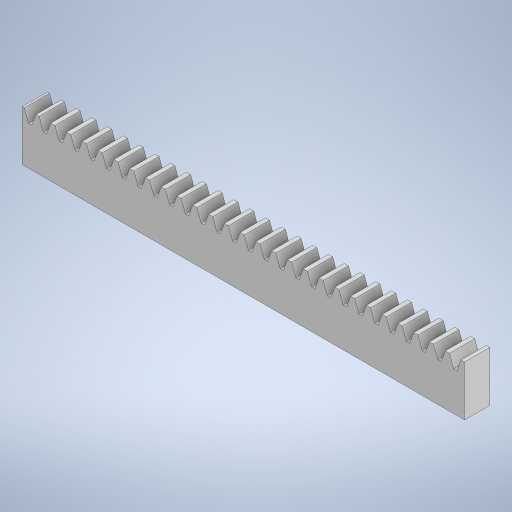
# Autodesk Inventor part: 래크수정
Saved by Autodesk Inventor 2024 (Build 280153000, 153)
## iProperties
Created: 2023-09-21
Part Number: 래크수정
Material: 일반
Document SubType Name: Modeling
Designer: user
Density: 1 g/cm^3
Appearance: 기본값
Author: user
Autodesk Inventor part; units mm, degrees
ref_plane "YZ Plane" through (0, 0, 0) normal (1, 0, 0) x (0, 1, 0)
ref_plane "XZ Plane" through (0, 0, 0) normal (0, 1, 0) x (-1, 0, 0)
ref_plane "XY Plane" through (0, 0, 0) normal (0, 0, 1) x (1, 0, 0)
sketch "스케치1" plane through (0, 0, 0) normal (0, 0, 1) x (1, 0, 0)
  line L0 (32.407, 33.8175) -> (32.407, 13.8175)
  line L1 (32.407, 13.8175) -> (-143.593, 13.8175)
  line L2 (-143.593, 13.8175) -> (-143.593, 33.8175)
  line L3 (-143.593, 29.3175) -> (32.407, 29.3175) construction
  line L4 (32.407, 31.8175) -> (-143.593, 31.8175) construction
  line L5 (-143.593, 29.8175) -> (32.407, 29.8175) construction
  line L6 (-140.453, 26.9927) -> (-140.453, 39.5951) construction
  line L7 (-137.313, 29.3175) -> (-137.313, 39.4326) construction
  line L8 (-142.751, 33.8175) -> (-141.1131, 29.3175)
  line L9 (-138.1551, 33.8175) -> (-139.7929, 29.3175)
  line L10 (-142.751, 33.8175) -> (-141.2951, 29.8175)
  line L11 (-138.1551, 33.8175) -> (-139.611, 29.8175)
  line L12 (-138.883, 31.8175) -> (-142.023, 31.8175) construction
  line L13 (-143.593, 33.8175) -> (-142.751, 33.8175)
  line L14 (-138.1551, 33.8175) -> (32.407, 33.8175)
  line L15 (-141.1131, 29.3175) -> (-139.7929, 29.3175)
  point P0 (0, 0)
  dimension "d0" = 176
  dimension "d1" = 20
  dimension "d6" = 2
  dimension "d8" = 6.28
  dimension "d10" = 20
  dimension "d11" = 3.14
  dimension "d12" = 3.14
  constraints: 32 end point, 12 point on line, 5 perpendicular, 3 parallel, 2 horizontal, 2 midpoint, 2 symmetric about line, 2 vertical, 1 collinear
  measures "d0" distance of L2.end L0.start
  measures "d1" distance of L0.start L0.end
  measures "d6" distance between parallel lines of L5 L4
  measures "d8" distance between parallel lines of L7 L2
  measures "d10" angle of L6 L8
  measures "d11" distance of L12.end L12.start
  measures "d12" distance between parallel lines of L2 L6
extrude "돌출1" add sketch "스케치1" against normal blind 10
sketch "스케치2" plane through (0, 0, 0) normal (0, 0, 1) x (1, 0, 0)
  line L0 (-259.941, 24.3877) -> (-259.941, 44.3877)
  line L1 (-256.801, 37.5629) -> (-256.801, 50.1653) construction
  line L2 (-253.661, 39.8877) -> (-253.661, 50.0028) construction
  line L3 (-259.0989, 44.3877) -> (-257.461, 39.8877)
  line L4 (-254.503, 44.3877) -> (-256.1409, 39.8877)
  line L5 (-259.0989, 44.3877) -> (-257.643, 40.3877)
  line L6 (-254.503, 44.3877) -> (-255.9589, 40.3877)
  line L7 (-255.231, 42.3877) -> (-258.371, 42.3877) construction
  line L8 (-259.941, 44.3877) -> (-259.0989, 44.3877)
  line L9 (-257.461, 39.8877) -> (-256.1409, 39.8877)
  line L10 (-143.5947, 29.322) -> (106.4053, 29.322) construction
  line L11 (-143.5963, 29.822) -> (106.4037, 29.822) construction
  line L12 (-140.4548, 26.9971) -> (-140.4548, 39.5996) construction
  line L13 (-137.4951, 29.322) -> (-137.4951, 39.3835) construction
  line L14 (-142.751, 33.8175) -> (-141.1148, 29.322)
  line L15 (-138.1585, 33.8175) -> (-139.7948, 29.322)
  line L16 (-138.8863, 31.822) -> (-142.0263, 31.822) construction
  line L17 (-143.593, 33.8175) -> (-142.751, 33.8175)
  line L18 (-141.1148, 29.322) -> (-139.7948, 29.322)
  line L19 (-137.306, 29.822) -> (112.694, 29.822) construction
  line L20 (-134.5388, 26.9971) -> (-134.5388, 39.5996) construction
  line L21 (-131.2358, 28.8786) -> (-131.2358, 38.9936) construction
  line L22 (-136.8351, 33.8175) -> (-135.1988, 29.322)
  line L23 (-132.2426, 33.8175) -> (-133.8788, 29.322)
  line L24 (-138.1585, 33.8175) -> (-136.8351, 33.8175)
  line L25 (-138.1551, 33.8175) -> (32.407, 33.8175) projected
  line L26 (-135.1988, 29.322) -> (-133.8788, 29.322)
  point P0 (0, 0)
  point P1 (-116.3479, 10.5702)
  dimension "d19" = 6.28
  dimension "d20" = 20
  dimension "d21" = 3.14
  dimension "d22" = 3.14
  dimension "d23" = 20
  dimension "d24" = 3.14
  dimension "d25" = 20
  dimension "d27" = 1.32
  dimension "d28" = 1.32
  dimension "d29" = 0.842
  dimension "d36" = 1.32
  dimension "d37" = 0.66
  constraints: 53 end point, 6 point on line, 6 vertical, 5 symmetric about line, 3 collinear, 2 horizontal, 2 midpoint
  measures "d19" distance between parallel lines of L2 L0
  measures "d20" angle of L1 L3
  measures "d21" distance of L7.end L7.start
  measures "d22" distance between parallel lines of L0 L1
  measures "d23" angle of L12 L14
  measures "d24" distance of L16.end L16.start
  measures "d25" angle of L20 L22
  measures "d27" distance of L22.start L25.start
  measures "d28" distance of L14.end L15.end
  measures "d29" distance of L17.start L14.start
  measures "d36" distance of L23.end L22.end
  measures "d37" distance from line of L25.start L13
extrude "돌출2" cut sketch "스케치2" against normal blind 10
pattern_linear "직사각형 패턴2" count 39 spacing 6.28 along (1, 0, 0) of "돌출2"
